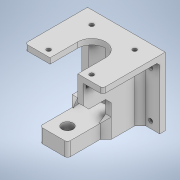
# Autodesk Inventor part: suporte barra motor
Saved by Autodesk Inventor 2022 (Build 260153000, 153)
## iProperties
Created: 2022-02-16
Part Number: suporte barra motor
Material: Genérico
Document SubType Name: Modeling
Designer: mathe
Density: 1 g/cm^3
Appearance: Padrão
Author: mathe
## iProperties of the stored document suporte barra motor_3DPrint.ipt
Created: 2022-02-18
Part Number: suporte barra motor_3DPrint
Material: Genérico
Document SubType Name: Modeling
Designer: mathe
Density: 1 g/cm^3
Appearance: Padrão
Author: mathe
Autodesk Inventor part; units mm, degrees
ref_plane "YZ Plane" through (0, 0, 0) normal (1, 0, 0) x (0, 1, 0)
ref_plane "XZ Plane" through (0, 0, 0) normal (0, 1, 0) x (-1, 0, 0)
ref_plane "XY Plane" through (0, 0, 0) normal (0, 0, 1) x (1, 0, 0)
sketch "Esboço1" plane through (0, 0, 0) normal (0, 0, 1) x (1, 0, 0)
  line L0 (0, 0) -> (56, 0)
  line L1 (56, 0) -> (56, 10)
  line L2 (56, 10) -> (0, 10)
  line L3 (0, 10) -> (0, 0)
  line L4 (18, 10) -> (38, 10)
  line L5 (38, 10) -> (38, 0)
  line L6 (38, 0) -> (18, 0)
  line L7 (18, 0) -> (18, 10)
  line L8 (18, 10) -> (38, 0) construction
  line L9 (38, 10) -> (18, 0) construction
  point P0 (28, 5)
  dimension "d0" = 56
  dimension "d1" = 10
  dimension "d2" = 20
  constraints: 20 end point, 4 parallel, 2 horizontal, 2 midpoint, 2 perpendicular, 1 point on line
  measures "d0" distance of L2.end L1.end
  measures "d1" distance of L1.end L0.end
  measures "d2" distance of L5.end L6.end
extrude "Extrusão1" add sketch "Esboço1" along normal blind 4 contours L3 L2 L7 L0 | L5 L2 L1 L0
extrude "Extrusão2" add sketch "Esboço1" along normal blind 52.426 contours L7 L2 L5 L0
sketch "Esboço2" plane through (0, 10, 0) normal (0, 1, 0) x (1, 0, 0)
  line L0 (38, -52.426) -> (18, -52.426) projected
  point P0 (0, 0)
  point P1 (28, -42.426)
  point P2 (33, -52.426)
  point P3 (23, -52.426)
  dimension "d24" = 10
  measures "d24" distance from line of L0 point (28, -42.426)
hole "Furo1" at (28, 10, 42.426) direction (0, -1, 0) diameter 8 end through all
sketch "Esboço3" plane through (0, 0, 4) normal (0, 0, 1) x (1, 0, 0)
  point P0 (0, 0)
  point P1 (6.5, 5)
  point P2 (49.5, 5)
hole "Furo2" at (6.5, 5, 4) at (49.5, 5, 4) direction (0, 0, -1) diameter 3 end through all
sketch "Esboço4" plane through (0, 10, 0) normal (0, 1, 0) x (1, 0, 0)
  line L0 (56, 0) -> (0, 0) projected
  line L1 (0, 0) -> (56, 0)
  line L2 (56, 0) -> (56, -25)
  line L3 (56, -25) -> (0, -25)
  line L4 (0, -25) -> (0, 0)
  dimension "d25" = 25
  constraints: 8 end point, 2 parallel, 1 horizontal, 1 perpendicular
  measures "d25" distance of L1.end L2.end
extrude "Extrusão3" add sketch "Esboço4" along normal blind 39
sketch "Esboço5" plane through (0, 49, 0) normal (0, 1, 0) x (1, 0, 0)
  line L0 (0, -25) -> (56, -25) projected
  circle A0 centre (28, -25) radius 10
  line L1 (38, -4) -> (38, -52.426) projected
  point P0 (0, 0)
  point P1 (38, -9)
  point P2 (38, -47.426)
  point P3 (38, -25)
  point P4 (18, -25)
  constraints: 1 centre point, 1 midpoint, 1 tangent
extrude "Extrusão4" cut sketch "Esboço5" against normal blind 22 contours A0 L0 picked at (30.9515, -23.4509)
sketch "Esboço6" plane through (0, 49, 0) normal (0, 1, 0) x (1, 0, 0)
  arc A0 (38, -25) -> (18, -25) centre (28, -25) ccw projected
  line L0 (18, -25) -> (18, -52.426) projected
  line L1 (0, -25) -> (18, -25)
  line L2 (18, -25) -> (18, -45)
  line L3 (18, -45) -> (0, -45)
  line L4 (0, -45) -> (0, -25)
  line L5 (38, -25) -> (38, -52.426) projected
  line L6 (56, -25) -> (38, -25)
  line L7 (38, -25) -> (38, -45)
  line L8 (38, -45) -> (56, -45)
  line L9 (56, -45) -> (56, -25)
  circle A1 centre (43.5, -9.5) radius 1.5
  circle A2 centre (12.5, -9.5) radius 1.5
  circle A3 centre (12.5, -40.5) radius 1.5
  circle A4 centre (43.5, -40.5) radius 1.5
  point P0 (0, 0)
  point P1 (18, -47.426)
  point P2 (38, -47.426)
  dimension "d30" = 15.5
  dimension "d31" = 15.5
  dimension "d32" = 15.5
  dimension "d33" = 15.5
  dimension "d34" = 20
  dimension "d37" = 3
  dimension "d38" = 3
  dimension "d39" = 3
  dimension "d40" = 3
  dimension "d87" = 15.5
  dimension "d88" = 15.5
  constraints: 16 end point, 4 centre point, 4 coincident, 4 parallel, 3 point on line, 2 horizontal, 2 perpendicular
  measures "d30" horizontal distance of point (43.5, -9.5) A0.centre
  measures "d31" horizontal distance of A0.centre point (43.5, -9.5)
  measures "d32" horizontal distance of point (12.5, -9.5) A0.centre
  measures "d33" horizontal distance of A0.centre point (12.5, -9.5)
  measures "d34" distance of L1.end L2.end
  measures "d37" diameter of A1
  measures "d38" diameter of A2
  measures "d39" diameter of A3
  measures "d40" diameter of A4
  measures "d87" distance from line of A3.centre L1
  measures "d88" distance from line of L6 A4.centre
extrude "Extrusão5" add sketch "Esboço6" against normal up to surface (22 mm away) contours L0 L3 L4 L1 | L6 L9 L8 L5 | A3 | A4
extrude "Extrusão6" cut sketch "Esboço6" against normal blind 20 contours A1 | A2 | A3 | A4
sketch "Esboço7" plane through (0, 0, 0) normal (-1, 0, 0) x (0, 0, 1)
  line L0 (4, 0) -> (4, 10) projected
  line L1 (45, 49) -> (45, 27) projected
  line L2 (4, 10) -> (45, 10)
  line L3 (45, 10) -> (45, 45)
  line L4 (45, 45) -> (4, 45)
  line L5 (4, 45) -> (4, 10)
  line L6 (0, 49) -> (45, 49) projected
  point P0 (0, 0)
  dimension "d43" = 4
  constraints: 8 end point, 2 parallel, 1 horizontal, 1 perpendicular, 1 point on line
  measures "d43" distance between parallel lines of L6 L4
extrude "Extrusão7" cut sketch "Esboço7" against normal blind 14
sketch "Esboço8" plane through (56, 0, 4) normal (1, 0, 0) x (0, 0, -1)
  line L0 (4, 0) -> (0, 0) projected
  line L1 (-41, 49) -> (-41, 27) projected
  line L2 (0, 0) -> (-41, 0)
  line L3 (-41, 0) -> (-41, 45)
  line L4 (-41, 45) -> (0, 45)
  line L5 (0, 45) -> (0, 0)
  line L6 (-41, 49) -> (4, 49) projected
  dimension "d46" = 4
  constraints: 8 end point, 2 parallel, 1 horizontal, 1 perpendicular, 1 point on line
  measures "d46" distance between parallel lines of L6 L4
extrude "Extrusão8" cut sketch "Esboço8" against normal blind 14
sketch "Esboço9" plane through (0, 27, 0) normal (0, 1, 0) x (1, 0, 0)
  line L0 (38, -25) -> (18, -25) projected
  circle A0 centre (28, -25) radius 10
  point P0 (0, 0)
  constraints: 1 centre point, 1 midpoint
extrude "Extrusão9" cut sketch "Esboço9" against normal up to surface (17 mm away) contours L0 A0 picked at (30.9515, -23.4509)
sketch "Esboço10" plane through (0, 10, 0) normal (0, -1, 0) x (1, 0, 0)
  line L0 (18, 25) -> (14, 25) projected
  line L1 (14, 4) -> (14, 9.5) projected
  line L2 (18, 25) -> (14, 25)
  line L3 (14, 25) -> (14, 4)
  line L4 (14, 4) -> (18, 4)
  line L5 (18, 4) -> (18, 25)
  line L6 (38, 25) -> (42, 25) projected
  line L7 (38, 4) -> (56, 4) projected
  line L8 (42, 25) -> (38, 25)
  line L9 (38, 25) -> (38, 4)
  line L10 (38, 4) -> (42, 4)
  line L11 (42, 4) -> (42, 25)
  point P0 (0, 0)
  constraints: 16 end point, 4 parallel, 2 horizontal, 2 perpendicular
extrude "Extrusão10" add sketch "Esboço10" along normal blind 10
chamfer "Chanfro2" distance 4 angle 45 8 edges at (42, 22.5, 4) (38, 5, 25) (18, 5, 25) (14, 22.5, 4) (16, 27, 25) (40, 27, 25) (40, 27, 45) (16, 27, 45)
fillet "Arredondamento1" radius 2 4 edges at (18, 5, 52.426) (38, 5, 52.426) (0, 47, 45) (56, 47, 45)
sketch "Esboço11" plane through (0, 0, 4) normal (0, 0, 1) x (1, 0, 0)
  circle A0 centre (6.5, 5) radius 1.5 projected
  line L0 (6.5, 5) -> (6.5, 38)
  point P0 (0, 0)
  point P1 (49.5, 38)
  dimension "d57" = 33
  constraints: 2 end point, 1 coincident, 1 vertical
  measures "d57" distance of L0.start L0.end
hole "Furo3" at (6.5, 38, 4) at (49.5, 38, 4) direction (0, 0, -1) diameter 3 end through all
chamfer "Chanfro3" distance 4 angle 45 2 edges at (39.9999, 10, 25) (16.0001, 10, 25)
sketch "Esboço12" plane through (42, 0, 4) normal (1, 0, 0) x (0, 0, -1)
  line L0 (-36.5, 45) -> (-34, 45)
  line L1 (-21, 49) -> (-41, 49) projected
  line L2 (-34, 45) -> (-34, 41)
  line L3 (-34, 41) -> (-39, 41)
  line L4 (-39, 41) -> (-39, 45)
  line L5 (-39, 45) -> (-36.5, 45)
  line L6 (-5.4522, 45) -> (-2.9522, 45)
  line L7 (-2.9522, 45) -> (-2.9522, 41)
  line L8 (-2.9522, 41) -> (-7.9522, 41)
  line L9 (-7.9522, 41) -> (-7.9522, 45)
  line L10 (-7.9522, 45) -> (-5.4522, 45)
  point P0 (4, 0)
  dimension "d68" = 2.5
  dimension "d69" = 4
  dimension "d70" = 5
  dimension "d71" = 2.5
  dimension "d72" = 4
  dimension "d73" = 5
  constraints: 20 end point, 8 perpendicular, 2 point on line, 1 parallel
  measures "d68" distance of L0.start L0.end
  measures "d69" distance of L0.end L2.end
  measures "d70" distance of L2.end L3.end
  measures "d71" distance of L6.start L6.end
  measures "d72" distance of L6.end L7.end
  measures "d73" distance of L7.end L8.end
extrude "Extrusão11" cut sketch "Esboço12" along normal mid plane 2
sketch "Esboço13" plane through (14, 0, 0) normal (-1, 0, 0) x (0, 0, 1)
  line L0 (9.5, 45) -> (40.5, 45) projected
  line L1 (40.5, 45) -> (38, 45)
  line L2 (38, 45) -> (38, 41)
  line L3 (38, 41) -> (43, 41)
  line L4 (43, 41) -> (43, 45)
  line L5 (43, 45) -> (40.5, 45)
  line L6 (9.5, 45) -> (7, 45)
  line L7 (7, 45) -> (7, 41)
  line L8 (7, 41) -> (12, 41)
  line L9 (12, 41) -> (12, 45)
  line L10 (12, 45) -> (9.5, 45)
  point P0 (0, 0)
  dimension "d76" = 2.5
  dimension "d77" = 4
  dimension "d78" = 5
  dimension "d79" = 2.5
  dimension "d80" = 4
  dimension "d81" = 5
  constraints: 20 end point, 8 perpendicular, 3 point on line
  measures "d76" distance of L0.end L1.end
  measures "d77" distance of L1.end L2.end
  measures "d78" distance of L2.end L3.end
  measures "d79" distance of L6.start L6.end
  measures "d80" distance of L6.end L7.end
  measures "d81" distance of L7.end L8.end
extrude "Extrusão12" cut sketch "Esboço13" along normal mid plane 2
chamfer "Chanfro4" distance 2 angle 45 2 edges at (5.0001, 45, 4) (51, 45, 4)
sketch "Esboço15" plane through (14, 31, 45) normal (0, 0, 1) x (1, 0, 0)
  line L0 (-3, 14) -> (0, 14) projected
  line L1 (4, -17) -> (4, -8) projected
  line L2 (0, 14) -> (4, 14)
  line L3 (4, -17) -> (0, -17)
  line L4 (0, -17) -> (0, 14)
  line L5 (4, 14) -> (14, 14)
  line L6 (14, 14) -> (14, -17)
  line L7 (14, -17) -> (4, -17)
  point P0 (-14, -31)
  constraints: 12 end point, 2 horizontal, 2 parallel, 1 perpendicular
extrude "Extrusão14" cut sketch "Esboço15" against normal up to surface (30 mm away)
chamfer "Chanfro5" distance 2 angle 45 2 edges at (21, 14, 15) (14, 29.5, 15)
